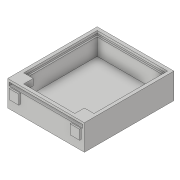
# Autodesk Inventor part: Electronics Container
Saved by Autodesk Inventor 2018.3 (Build 223284000, 284)
## iProperties
Created: 2019-01-09
Part Number: Electronics Container
Material: Generic
Document SubType Name: Modeling
Designer: aye06091
Mass: 43.4161 g
Surface Area: 302.419 cm^2
Volume: 43.4161 cm^3
Density: 1 g/cm^3
Appearance: Default
Author: aye06091
Autodesk Inventor part; units mm, degrees
ref_plane "YZ Plane" through (0, 0, 0) normal (1, 0, 0) x (0, 1, 0)
ref_plane "XZ Plane" through (0, 0, 0) normal (0, 1, 0) x (-1, 0, 0)
ref_plane "XY Plane" through (0, 0, 0) normal (0, 0, 1) x (1, 0, 0)
sketch "Sketch1" plane through (0, 0, 0) normal (0, 0, 1) x (1, 0, 0)
  line L0 (0, 0) -> (76.2, 0)
  line L1 (76.2, 0) -> (76.2, -25.4)
  line L2 (76.2, -25.4) -> (0, -25.4)
  line L3 (0, -25.4) -> (0, 0)
  dimension "d0" = 76.2
  dimension "d1" = 25.4
  constraints: 8 end point, 2 parallel, 1 horizontal, 1 perpendicular
  measures "d0" distance of L1.end L2.end
  measures "d1" distance of L2.end L0.start
extrude "Extrusion1" add sketch "Sketch1" against normal blind 88.9
sketch "Sketch2" plane through (0, 0, 0) normal (0, 1, 0) x (1, 0, 0)
  line L0 (0, 0) -> (76.2, 0) projected
  line L1 (76.2, 0) -> (76.2, 88.9) projected
  line L2 (0, 88.9) -> (76.2, 88.9) projected
  line L3 (0, 0) -> (0, 88.9) projected
  line L4 (3.175, 3.175) -> (73.025, 3.175)
  line L5 (73.025, 3.175) -> (73.025, 85.725)
  line L6 (73.025, 85.725) -> (3.175, 85.725)
  line L7 (3.175, 85.725) -> (3.175, 3.175)
  dimension "d4" = 3.175
  dimension "d5" = 3.175
  dimension "d6" = 3.175
  dimension "d7" = 3.175
  constraints: 8 end point, 2 parallel, 1 horizontal, 1 perpendicular
  measures "d4" distance between parallel lines of L3 L7
  measures "d5" distance between parallel lines of L0 L4
  measures "d6" distance between parallel lines of L1 L5
  measures "d7" distance between parallel lines of L2 L6
extrude "Extrusion2" cut sketch "Sketch2" against normal blind 22.225 contours L7 L6 L5 L4
sketch "Sketch3" plane through (0, 0, 0) normal (0, 0, 1) x (1, 0, 0)
  line L0 (0, -25.4) -> (0, 0) projected
  line L1 (76.2, 0) -> (76.2, -25.4) projected
  line L2 (0, -25.4) -> (0, 0) projected
  line L3 (76.2, 0) -> (76.2, -25.4) projected
  line L4 (1.5875, -2.3041) -> (74.6125, -2.3041)
  line L5 (74.6125, -2.3041) -> (74.6125, -5.4791)
  line L6 (74.6125, -5.4791) -> (1.5875, -5.4791)
  line L7 (1.5875, -5.4791) -> (1.5875, -2.3041)
  dimension "d46" = 3.175
  dimension "d47" = 1.5875
  dimension "d49" = 1.5875
  constraints: 8 end point, 2 parallel, 1 horizontal, 1 perpendicular
  measures "d46" distance between parallel lines of L6 L4
  measures "d47" distance between parallel lines of L0 L7
  measures "d49" distance between parallel lines of L1 L5
extrude "Extrusion3" cut sketch "Sketch3" against normal blind 87.3125
sketch "Sketch5" plane through (0, 0, 0) normal (0, 1, 0) x (1, 0, 0)
  line L0 (3.175, 3.175) -> (3.175, 85.725) projected
  line L1 (3.175, 3.175) -> (12.7, 3.175)
  line L2 (12.7, 3.175) -> (12.7, 12.7)
  line L3 (12.7, 12.7) -> (3.175, 12.7)
  line L4 (3.175, 12.7) -> (3.175, 3.175)
  line L5 (73.025, 3.175) -> (63.5, 3.175)
  line L6 (63.5, 3.175) -> (63.5, 12.7)
  line L7 (63.5, 12.7) -> (73.025, 12.7)
  line L8 (73.025, 12.7) -> (73.025, 3.175)
  dimension "d64" = 9.525
  dimension "d67" = 9.525
  dimension "d68" = 9.525
  dimension "d69" = 9.525
  constraints: 16 end point, 4 parallel, 2 horizontal, 2 perpendicular
  measures "d64" distance of L6.end L7.end
  measures "d67" distance of L2.end L3.end
  measures "d68" distance of L1.end L2.end
  measures "d69" distance of L5.end L6.end
extrude "Extrusion4" add sketch "Sketch5" against normal blind 6.35
sketch "Sketch6" plane through (0, 0, 0) normal (0, 0, 1) x (1, 0, 0)
  line L0 (12.6756, -6.3523) -> (3.1506, -6.3523)
  line L1 (3.1506, -6.3523) -> (3.1506, -15.8773)
  line L2 (3.1506, -15.8773) -> (12.6756, -15.8773)
  line L3 (12.6756, -15.8773) -> (12.6756, -6.3523)
  line L4 (63.5241, -6.3523) -> (73.0491, -6.3523)
  line L5 (73.0491, -6.3523) -> (73.0491, -15.8773)
  line L6 (73.0491, -15.8773) -> (63.5241, -15.8773)
  line L7 (63.5241, -15.8773) -> (63.5241, -6.3523)
  dimension "d70" = 9.525
  dimension "d71" = 9.525
  dimension "d72" = 9.525
  dimension "d73" = 9.525
  constraints: 16 end point, 4 parallel, 2 horizontal, 2 perpendicular, 2 point on line
  measures "d70" distance of L0.start L0.end
  measures "d71" distance of L2.end L0.start
  measures "d72" distance of L6.end L4.start
  measures "d73" distance of L4.start L4.end
extrude "Extrusion5" add sketch "Sketch6" along normal blind 1.5875
equation "\"d49\" = d47"
equation "\"d65\" = d62"
equation "\"d73\" = d71"
equation "\"d62\" = 6.35"
body "Solid1"
